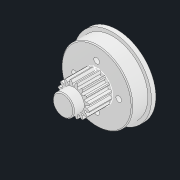
# Autodesk Inventor part: s-assy-sun_gear
Saved by Autodesk Inventor 2022 (Build 260153000, 153)
## iProperties
Created: 2021-07-12
Part Number: s-assy-sun_gear
Material: ABS プラスチック
Document SubType Name: Modeling
Designer: yuta0
Density: 1.06 g/cm^3
Appearance: 滑らか - 白
購入先: 印刷
在庫数: 0.0
Author: yuta0
Autodesk Inventor part; units mm, degrees
ref_plane "YZ Plane" through (0, 0, 0) normal (1, 0, 0) x (0, 1, 0)
ref_plane "XZ Plane" through (0, 0, 0) normal (0, 1, 0) x (-1, 0, 0)
ref_plane "XY Plane" through (0, 0, 0) normal (0, 0, 1) x (1, 0, 0)
sketch "スケッチ1" plane through (0, 0, 0) normal (1, 0, 0) x (0, 1, 0)
  line L0 (22, 0) -> (22, 2.5)
  line L1 (22, 2.5) -> (20, 2.5)
  line L2 (20, 2.5) -> (20, 11.5)
  line L3 (20, 11.5) -> (0, 11.5)
  line L4 (0, 11.5) -> (0, 0)
  line L5 (0, 0) -> (22, 0)
  dimension "d0" = 20
  dimension "d1" = 9
  dimension "d2" = 2.5
  dimension "d3" = 2
  constraints: 12 end point, 5 perpendicular, 1 vertical
  measures "d0" distance of L2.end L3.end
  measures "d1" distance of L1.end L2.end
  measures "d2" distance of L0.start L0.end
  measures "d3" distance of L0.end L1.end
revolve "回転1" add sketch "スケッチ1" angle 360 about axis through (0, 0, 11.5) along (0, 0, -1)
sketch "スケッチ2" plane through (0, 0, 11.5) normal (0, 0, 1) x (1, 0, 0)
  spline S0 degree 3 poles (-1.4856, 8.8744) (-1.4402, 8.8245) (-1.3495, 8.7245) (-1.222, 8.5671) (-1.1015, 8.4042) (-0.9897, 8.2353) (-0.8878, 8.0602) (-0.8127, 7.9089) (-0.7601, 7.7845) (-0.7252, 7.6895) (-0.6947, 7.5928) (-0.6821, 7.5264) (-0.6758, 7.4933) knots 0 0 0 0 0.020249 0.040498 0.060747 0.080996 0.101243 0.12149 0.131614 0.141739 0.151862 0.161982 0.161982 0.161982 0.161982
  spline S1 degree 3 poles (-0.6758, 7.4933) (-0.6737, 7.4405) (-0.6706, 7.3613) (-0.6573, 7.2564) (-0.6428, 7.1785) (-0.6232, 7.1017) (-0.5986, 7.0263) (-0.5682, 6.953) (-0.5302, 6.8834) (-0.4861, 6.8175) (-0.434, 6.7575) (-0.3745, 6.7049) (-0.3077, 6.6618) (-0.2472, 6.6351) (-0.197, 6.6184) (-0.158, 6.611) (-0.1189, 6.6045) (-0.066, 6.6033) (0, 6.6042) (0.066, 6.6033) (0.1189, 6.6045) (0.158, 6.611) (0.197, 6.6184) (0.2472, 6.6351) (0.3077, 6.6618) (0.3745, 6.7049) (0.434, 6.7575) (0.4861, 6.8175) (0.5302, 6.8834) (0.5682, 6.953) (0.5986, 7.0263) (0.6232, 7.1017) (0.6428, 7.1785) (0.6573, 7.2564) (0.6706, 7.3613) (0.6737, 7.4405) (0.6758, 7.4933) knots 0 0 0 0 0.015842 0.023764 0.031687 0.03961 0.04753 0.055453 0.063374 0.071292 0.07921 0.087128 0.095042 0.102956 0.106917 0.110878 0.11484 0.118801 0.126724 0.134647 0.138608 0.14257 0.14653 0.150492 0.158406 0.16632 0.174238 0.182155 0.190073 0.197995 0.205917 0.213838 0.221761 0.229684 0.237606 0.253448 0.253448 0.253448 0.253448
  spline S2 degree 3 poles (0.6758, 7.4933) (0.6821, 7.5264) (0.6947, 7.5928) (0.7252, 7.6895) (0.7601, 7.7845) (0.8127, 7.9089) (0.8878, 8.0602) (0.9897, 8.2353) (1.1015, 8.4042) (1.222, 8.5671) (1.3495, 8.7245) (1.4402, 8.8245) (1.4856, 8.8744) knots 0 0 0 0 0.010119 0.020243 0.030367 0.040492 0.060738 0.080986 0.101235 0.121483 0.141733 0.161982 0.161982 0.161982 0.161982
  circle A0 centre (0, 0) radius 6.6038 construction
  circle A1 centre (0, 0) radius 7.5175 construction
  circle A2 centre (0, 0) radius 8 construction
  circle A3 centre (0, 0) radius 8.9979
  point P0 (-1.3509, 8.7233)
  point P1 (-1.2231, 8.5662)
  point P2 (-1.1029, 8.4032)
  point P3 (-0.9914, 8.2342)
  point P4 (-0.8898, 8.0591)
  point P5 (-0.8002, 7.8775)
  point P6 (-0.7608, 7.7842)
  point P7 (-0.7259, 7.6892)
  point P8 (-0.6966, 7.5923)
  point P9 (-0.6665, 7.3351)
  point P10 (-0.6566, 7.2565)
  point P11 (-0.642, 7.1787)
  point P12 (-0.6223, 7.1019)
  point P13 (-0.5977, 7.0266)
  point P14 (-0.567, 6.9536)
  point P15 (-0.5292, 6.884)
  point P16 (-0.4848, 6.8184)
  point P17 (-0.4328, 6.7587)
  point P18 (-0.3733, 6.7065)
  point P19 (-0.3067, 6.6636)
  point P20 (-0.2345, 6.6313)
  point P21 (-0.1968, 6.6192)
  point P22 (-0.158, 6.6112)
  point P23 (-0.1188, 6.6054)
  point P24 (-0.0792, 6.6037)
  point P25 (0, 6.6038)
  point P26 (0.0792, 6.6037)
  point P27 (0.1188, 6.6054)
  point P28 (0.158, 6.6112)
  point P29 (0.1968, 6.6192)
  point P30 (0.2345, 6.6313)
  point P31 (0.3067, 6.6636)
  point P32 (0.3733, 6.7065)
  point P33 (0.4328, 6.7587)
  point P34 (0.4848, 6.8184)
  point P35 (0.5292, 6.884)
  point P36 (0.567, 6.9536)
  point P37 (0.5977, 7.0266)
  point P38 (0.6223, 7.1019)
  point P39 (0.642, 7.1787)
  point P40 (0.6566, 7.2565)
  point P41 (0.6665, 7.3351)
  point P42 (0.6966, 7.5923)
  point P43 (0.7259, 7.6892)
  point P44 (0.7608, 7.7842)
  point P45 (0.8002, 7.8775)
  point P46 (0.8898, 8.0591)
  point P47 (0.9914, 8.2342)
  point P48 (1.1029, 8.4032)
  point P49 (1.2231, 8.5662)
  point P50 (1.3509, 8.7233)
  constraints: 4 centre point, 2 point on circle, 117 other
extrude "押し出し1" add sketch "スケッチ2" along normal blind 13
extrude "押し出し3" cut sketch "スケッチ2" along normal through all contours A3 S2 S1 S0 picked at (-0.1735, 8.2566)
pattern_circular "円形状パターン1" count 16 over 360 about axis through (0, 0, -10) along (0, 0, 1) of "押し出し3"
sketch "スケッチ3" plane through (0, 0, 24.5) normal (0, 0, 1) x (1, 0, 0)
  circle A0 centre (0, 0) radius 6
  dimension "d7" = 12
  constraints: 1 centre point, 1 coincident
  measures "d7" diameter of A0
extrude "押し出し2" add sketch "スケッチ3" along normal blind 6
chamfer "面取り1" distance 0.5 angle 45 2 edges at (-6, 0, 30.5) (0, -20, 11.5)
sketch "スケッチ4" plane through (0, 0, 11.5) normal (0, 0, 1) x (1, 0, 0)
  circle A0 centre (0, 0) radius 12.5
  point P0 (0, 0)
  point P1 (0, 12.5)
  point P2 (-12.5, 0)
  point P3 (0, -12.5)
  point P4 (12.5, 0)
  dimension "d13" = 25
  dimension "d16" = 360
  constraints: 1 coincident, 1 vertical alignment, 7 other
hole "穴1" at (0, 12.5, 11.5) at (-12.5, 0, 11.5) at (0, -12.5, 11.5) at (12.5, 0, 11.5) direction (0, 0, -1) diameter 3.2 end through all clearance for "Flat Head Machine Screw" size "M3" standard "Ansi Metric M Profile"
